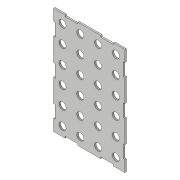
# Autodesk Inventor part: Base_modulos
Saved by Autodesk Inventor 2017 (Build 210142000, 142)
## iProperties
Created: 2017-06-21
Part Number: Base_modulos
Material: Generic
Document SubType Name: Modeling
Designer: Butri
Density: 1 g/cm^3
Appearance: Default
Author: Butri
Autodesk Inventor part; units mm, degrees
ref_plane "YZ Plane" through (0, 0, 0) normal (1, 0, 0) x (0, 1, 0)
ref_plane "XZ Plane" through (0, 0, 0) normal (0, 1, 0) x (-1, 0, 0)
ref_plane "XY Plane" through (0, 0, 0) normal (0, 0, 1) x (1, 0, 0)
sketch "Sketch1" plane through (0, 0, 0) normal (0, 1, 0) x (-1, 0, 0)
  line L0 (140, 210) -> (-140, 210)
  line L1 (-140, 210) -> (-140, -210)
  line L2 (-140, -210) -> (140, -210)
  line L3 (140, -210) -> (140, 210)
  line L4 (140, 210) -> (-140, -210) construction
  line L5 (-140, 210) -> (140, -210) construction
  point P0 (0, 0)
  dimension "d0" = 280
  dimension "d1" = 420
  constraints: 12 end point, 2 midpoint, 2 parallel, 1 horizontal, 1 perpendicular
  measures "d0" distance of L2.end L1.end
  measures "d1" distance of L1.end L0.end
extrude "Extrusion1" add sketch "Sketch1" along normal blind 6
sketch "Sketch2" plane through (0, 6, 0) normal (0, 1, 0) x (1, 0, 0)
  circle A0 centre (105, -175) radius 14
  line L0 (-140, -210) -> (140, -210) projected
  line L1 (140, -210) -> (140, 210) projected
  point P0 (0, 0)
  dimension "d4" = 28
  dimension "d5" = 35
  dimension "d6" = 35
  constraints: 1 centre point
  measures "d4" diameter of A0
  measures "d5" distance from line of L0 A0.centre
  measures "d6" distance from line of L1 A0.centre
extrude "Extrusion2" cut sketch "Sketch2" against normal blind 6
sketch "Sketch3" plane through (0, 6, 0) normal (0, 1, 0) x (1, 0, 0)
  circle A0 centre (135, -205) radius 1.75
  line L0 (-140, -210) -> (140, -210) projected
  line L1 (140, -210) -> (140, 210) projected
  circle A1 centre (75.5, -205) radius 1.75
  circle A2 centre (135, -145.5) radius 1.75
  circle A3 centre (75.5, -145.5) radius 1.75
  point P0 (0, 0)
  dimension "d15" = 3.5
  dimension "d16" = 5
  dimension "d17" = 5
  dimension "d18" = 3.5
  dimension "d19" = 5
  dimension "d20" = 59.5
  dimension "d21" = 3.5
  dimension "d22" = 5
  dimension "d23" = 59.5
  dimension "d24" = 3.5
  dimension "d25" = 59.5
  dimension "d26" = 59.5
  constraints: 4 centre point
  measures "d15" diameter of A0
  measures "d16" distance from line of L0 A0.centre
  measures "d17" distance from line of L1 A0.centre
  measures "d18" diameter of A1
  measures "d19" distance from line of L0 A1.centre
  measures "d20" distance of A1.centre A0.centre
  measures "d21" diameter of A2
  measures "d22" distance from line of L1 A2.centre
  measures "d23" distance of A0.centre A2.centre
  measures "d24" diameter of A3
  measures "d25" distance of A2.centre A3.centre
  measures "d26" distance of A1.centre A3.centre
pattern_linear "Rectangular Pattern1" count 6 spacing 70 along (0, 0, -1) count 4 spacing 70 along (-1, 0, 0) of "Extrusion2"
sketch "Sketch4" plane through (0, 6, 0) normal (0, 1, 0) x (1, 0, 0)
  line L0 (140, -210) -> (140, 210) projected
  line L1 (140, -25) -> (134, -25)
  line L2 (134, -25) -> (134, 25)
  line L3 (134, 25) -> (140, 25)
  line L4 (140, 25) -> (140, -25)
  line L5 (0, -210) -> (0, 210) construction
  line L6 (140, -165) -> (134, -165)
  line L7 (134, -165) -> (134, -115)
  line L8 (134, -115) -> (140, -115)
  line L9 (140, -115) -> (140, -165)
  line L10 (-140, -210) -> (140, -210) projected
  line L11 (140, 115) -> (134, 115)
  line L12 (134, 115) -> (134, 165)
  line L13 (134, 165) -> (140, 165)
  line L14 (140, 165) -> (140, 115)
  line L15 (140, 210) -> (-140, 210) projected
  line L16 (-140, -25) -> (-134, -25)
  line L17 (-134, -25) -> (-134, 25)
  line L18 (-134, 25) -> (-140, 25)
  line L19 (-140, 25) -> (-140, -25)
  line L20 (-140, -165) -> (-134, -165)
  line L21 (-134, -165) -> (-134, -115)
  line L22 (-134, -115) -> (-140, -115)
  line L23 (-140, -115) -> (-140, -165)
  line L24 (-140, 115) -> (-134, 115)
  line L25 (-134, 115) -> (-134, 165)
  line L26 (-134, 165) -> (-140, 165)
  line L27 (-140, 165) -> (-140, 115)
  line L28 (-95, -210) -> (-45, -210)
  line L29 (-45, -210) -> (-45, -204)
  line L30 (-45, -204) -> (-95, -204)
  line L31 (-95, -204) -> (-95, -210)
  line L32 (-140, 210) -> (-140, -210) projected
  line L33 (45, -210) -> (95, -210)
  line L34 (95, -210) -> (95, -204)
  line L35 (95, -204) -> (45, -204)
  line L36 (45, -204) -> (45, -210)
  line L37 (-140, 0) -> (140, 0) construction
  line L38 (-95, 210) -> (-45, 210)
  line L39 (-45, 210) -> (-45, 204)
  line L40 (-45, 204) -> (-95, 204)
  line L41 (-95, 204) -> (-95, 210)
  line L42 (45, 210) -> (95, 210)
  line L43 (95, 210) -> (95, 204)
  line L44 (95, 204) -> (45, 204)
  line L45 (45, 204) -> (45, 210)
  point P0 (0, 0)
  dimension "d35" = 6
  dimension "d36" = 50
  dimension "d37" = 6
  dimension "d38" = 50
  dimension "d39" = 45
  dimension "d40" = 6
  dimension "d41" = 50
  dimension "d42" = 45
  dimension "d43" = 50
  dimension "d44" = 6
  dimension "d45" = 45
  dimension "d46" = 50
  dimension "d47" = 6
  dimension "d48" = 45
  constraints: 84 end point, 21 symmetric about line, 10 parallel, 6 perpendicular, 5 horizontal, 5 point on line, 2 midpoint, 1 vertical
  measures "d35" distance of L2.end L3.end
  measures "d36" distance of L1.end L2.end
  measures "d37" distance of L7.end L8.end
  measures "d38" distance of L6.end L7.end
  measures "d39" distance between parallel lines of L10 L6
  measures "d40" distance of L12.end L13.end
  measures "d41" distance of L11.end L12.end
  measures "d42" distance between parallel lines of L15 L13
  measures "d43" distance of L30.end L29.end
  measures "d44" distance of L29.end L28.end
  measures "d45" distance between parallel lines of L32 L31
  measures "d46" distance of L35.end L34.end
  measures "d47" distance of L34.end L33.end
  measures "d48" distance between parallel lines of L0 L34
extrude "Extrusion4" cut sketch "Sketch4" against normal blind 6 contours L6 L7 L8 L0 | L10 L36 L35 L34 | L1 L2 L3 L0 | L10 L31 L30 L29 | L11 L12 L13 L0 | L23 L22 L21 L20 | L43 L44 L45 L15 | L19 L18 L17 L16 | L39 L40 L41 L15 | L27 L26 L25 L24
equation "\"d17\" = d16"
equation "\"d19\" = d16"
equation "\"d22\" = d16"
equation "\"d23\" = d20"
equation "\"d25\" = d20"
equation "\"d26\" = d20"
body "Solid1"
